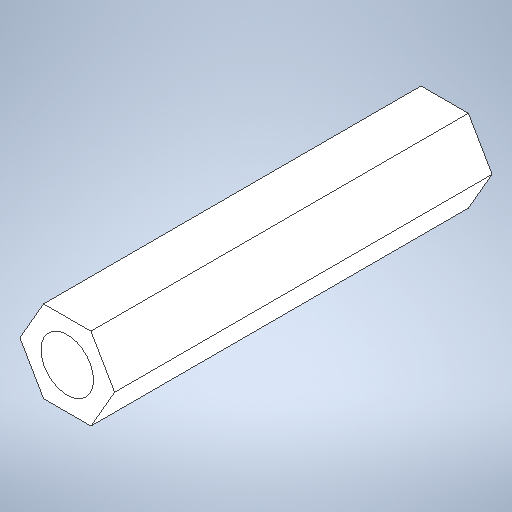
# Autodesk Inventor part: キャスタスペーサ
Saved by Autodesk Inventor 2026.2 (Build 302298010, 298A)
## iProperties
Created: 2026-05-06
Part Number: キャスタスペーサ
Material: 一般
Document SubType Name: Modeling
Designer: Yagis
Density: 1 g/cm^3
Appearance: 既定
Author: Yagis
Autodesk Inventor part; units mm, degrees
ref_plane "YZ Plane" through (0, 0, 0) normal (1, 0, 0) x (0, 1, 0)
ref_plane "XZ Plane" through (0, 0, 0) normal (0, 1, 0) x (-1, 0, 0)
ref_plane "XY Plane" through (0, 0, 0) normal (0, 0, 1) x (1, 0, 0)
sketch "スケッチ1" plane through (0, 0, 0) normal (0, 0, 1) x (1, 0, 0)
  line L0 (1.4411, 2.5013) -> (2.8868, 0.0026)
  line L1 (2.8868, 0.0026) -> (1.4456, -2.4987)
  line L2 (1.4456, -2.4987) -> (-1.4411, -2.5013)
  line L3 (-1.4411, -2.5013) -> (-2.8868, -0.0026)
  line L4 (-2.8868, -0.0026) -> (-1.4456, 2.4987)
  line L5 (-1.4456, 2.4987) -> (1.4411, 2.5013)
  circle A0 centre (0, 0) radius 1.6
  dimension "d0" = 3.2
  dimension "d1" = 5
  constraints: 12 end point, 2 coincident, 1 centre point, 13 other
  measures "d0" diameter of A0
  measures "d1" distance between parallel lines of L2 L5
extrude "押し出し1" add sketch "スケッチ1" along normal blind 23
